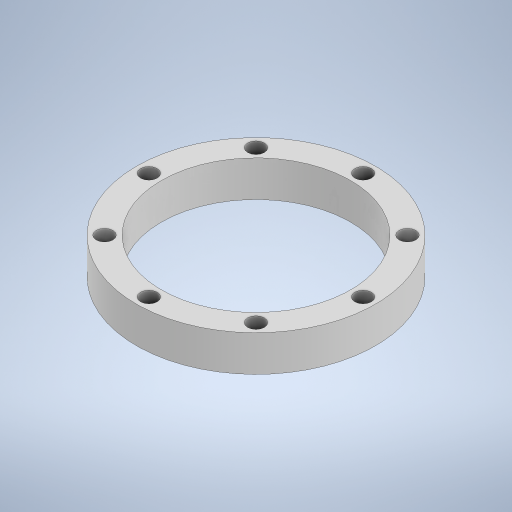
# Autodesk Inventor part: Bell_KoloFormaGora
Saved by Autodesk Inventor 2023 (Build 270158000, 158)
## iProperties
Created: 2023-05-03
Part Number: Bell_KoloFormaGora
Material: Ogólny
Document SubType Name: Modeling
Designer: julia
Density: 1 g/cm^3
Appearance: Domyślna
Author: julia
Autodesk Inventor part; units mm, degrees
ref_plane "YZ Plane" through (0, 0, 0) normal (1, 0, 0) x (0, 1, 0)
ref_plane "XZ Plane" through (0, 0, 0) normal (0, 1, 0) x (-1, 0, 0)
ref_plane "XY Plane" through (0, 0, 0) normal (0, 0, 1) x (1, 0, 0)
sketch "Szkic1" plane through (0, 0, 0) normal (0, 1, 0) x (-1, 0, 0)
  circle A0 centre (0, 0) radius 21
  circle A1 centre (0, 0) radius 26.5
  circle A2 centre (16.7938, 16.7938) radius 1.85
  circle A3 centre (0, 23.75) radius 1.85
  circle A4 centre (-16.7938, 16.7938) radius 1.85
  circle A5 centre (-23.75, 0) radius 1.85
  circle A6 centre (-16.7938, -16.7938) radius 1.85
  circle A7 centre (0, -23.75) radius 1.85
  circle A8 centre (16.7938, -16.7938) radius 1.85
  circle A9 centre (23.75, 0) radius 1.85
  line L0 (0, 21) -> (0, 26.5)
  dimension "d0" = 42
  dimension "d8" = 53
  dimension "d1" = 3.7
  dimension "d4" = 360
  constraints: 8 centre point, 3 coincident, 2 end point, 2 vertical alignment, 1 midpoint, 1 vertical, 21 other
  measures "d1" diameter of A2
extrude "Wyciągnięcie proste1" add sketch "Szkic1" along normal blind 8
